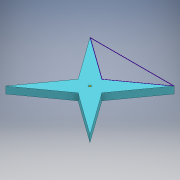
# Autodesk Inventor part: Dispensing Gear
Saved by Autodesk Inventor 2017 (Build 210142000, 142)
## iProperties
Created: 2018-12-12
Part Number: Dispensing Gear
Material: Generic
Document SubType Name: Modeling
Designer: Matt
Density: 1 g/cm^3
Appearance: Cadet Blue
Author: Matt
Autodesk Inventor part; units mm, degrees
ref_plane "YZ Plane" through (0, 0, 0) normal (1, 0, 0) x (0, 1, 0)
ref_plane "XZ Plane" through (0, 0, 0) normal (0, 1, 0) x (-1, 0, 0)
ref_plane "XY Plane" through (0, 0, 0) normal (0, 0, 1) x (1, 0, 0)
sketch "Sketch1" plane through (0, 0, 0) normal (0, 0, 1) x (1, 0, 0)
  arc A0 (-1.473, 2.02) -> (1.473, 2.02) centre (0, 0) ccw
  line L0 (0, 2.5) -> (0, 2.02)
  line L1 (0, 2.02) -> (1.473, 2.02)
  line L2 (0, 2.02) -> (-1.473, 2.02)
  line L3 (0, 0) -> (125, 0) construction
  line L4 (88.3883, 88.3883) -> (0.0691, 24.9999)
  line L5 (-88.2502, 88.3883) -> (0.0691, 24.9999)
  line L6 (0.0691, 24.9999) -> (-88.2502, 88.3883)
  line L7 (88.3883, 88.3883) -> (0.0691, 24.9999)
  line L8 (25, 0) -> (88.3883, 88.3883)
  line L9 (-24.9987, 0.2597) -> (-88.2502, 88.3883)
  line L10 (0, 0) -> (7.0052, 0)
  line L11 (88.3883, -88.3883) -> (0.0691, -24.9999)
  line L12 (-88.2502, -88.3883) -> (0.0691, -24.9999)
  line L13 (25, 0) -> (88.3883, -88.3883)
  line L14 (-24.9987, -0.2597) -> (-88.2502, -88.3883)
  line L15 (0.0691, -24.9999) -> (-88.2502, -88.3883)
  line L16 (-88.2502, -88.3883) -> (-24.9987, -0.2597)
  line L17 (88.3883, -88.3883) -> (0.0691, -24.9999)
  line L18 (88.3883, -88.3883) -> (25, 0)
  line L19 (88.3883, -88.3883) -> (0.0691, -24.9999)
  line L20 (0.0691, -24.9999) -> (-88.2502, -88.3883)
  line L21 (-88.2502, -88.3883) -> (-24.9987, -0.2597)
  line L22 (-24.9987, -0.2597) -> (-24.8122, 0)
  line L23 (-24.8122, 0) -> (-24.9987, 0.2597)
  dimension "d0" = 5
  dimension "d1" = 0.48
  dimension "d3" = 125
  constraints: 48 end point, 7 collinear, 4 symmetric about line, 3 perpendicular, 3 point on line, 2 coincident, 2 point on circle, 1 centre point, 1 horizontal, 1 vertical
  measures "d0" diameter of A0
  measures "d1" distance of L0.start L0.end
  measures "d3" distance of L3.start L4.start
extrude "Extrusion1" add sketch "Sketch1" along normal blind 14.5
sketch "Sketch2" plane through (0, 0, 14.5) normal (0, 0, 1) x (1, 0, 0)
  line L0 (0.0691, 24.9999) -> (-88.2502, 88.3883) projected
  line L1 (0.0691, 24.9999) -> (-88.2502, 88.3883)
  line L2 (88.3883, 88.3883) -> (0.0691, 24.9999) projected
  line L3 (-88.2502, 88.3883) -> (88.3883, 88.3883)
  line L4 (88.3883, 88.3883) -> (0.0691, 24.9999)
  point P0 (0, 0)
  constraints: 6 end point, 2 collinear, 1 horizontal
body "Solid1"
